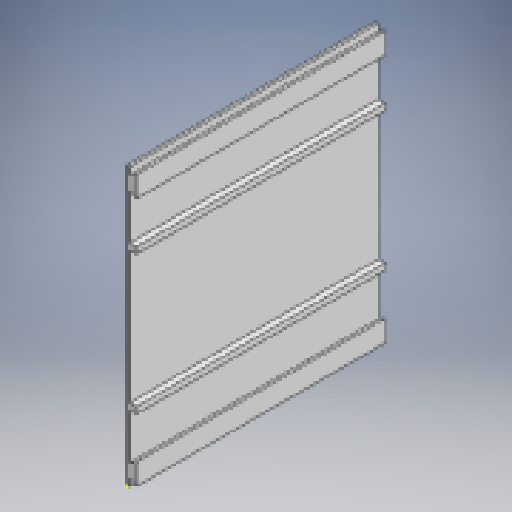
# Autodesk Inventor part: side
Saved by Autodesk Inventor 2025.2 (Build 292293000, 293)
## iProperties
Created: 2025-02-22
Part Number: side
Material: Generic
Document SubType Name: Modeling
Designer: email
Density: 1 g/cm^3
Appearance: Default
Author: email
Autodesk Inventor part; units mm, degrees
ref_plane "YZ Plane" through (0, 0, 0) normal (1, 0, 0) x (0, 1, 0)
ref_plane "XZ Plane" through (0, 0, 0) normal (0, 1, 0) x (-1, 0, 0)
ref_plane "XY Plane" through (0, 0, 0) normal (0, 0, 1) x (1, 0, 0)
sketch "Sketch1" plane through (0, 0, 0) normal (0, 0, 1) x (1, 0, 0)
  line L0 (0, 0) -> (0, 100)
  line L1 (0, 100) -> (1, 100)
  line L2 (1, 100) -> (1, 97.5)
  line L3 (1, 97.5) -> (3.5, 99)
  line L4 (3.5, 99) -> (3.5, 91)
  line L5 (3.5, 91) -> (1, 92.5)
  line L6 (1, 92.5) -> (1, 7.5)
  line L7 (1, 7.5) -> (3.5, 9)
  line L8 (3.5, 9) -> (3.5, 1)
  line L9 (3.5, 1) -> (1, 2.5)
  line L10 (1, 2.5) -> (1, 0)
  line L11 (1, 0) -> (0, 0)
  line L12 (1, 76.25) -> (3.5, 76.25)
  line L13 (3.5, 76.25) -> (3.5, 73.75)
  line L14 (3.5, 73.75) -> (1, 73.75)
  line L15 (1, 73.75) -> (1, 76.25)
  line L16 (1, 23.75) -> (3.5, 23.75)
  line L17 (3.5, 23.75) -> (3.5, 26.25)
  line L18 (3.5, 26.25) -> (1, 26.25)
  line L19 (1, 26.25) -> (1, 23.75)
  line L20 (3.4, 98.8234) -> (0.9, 97.3234)
  line L21 (0.9, 97.3234) -> (0.9, 99.9)
  line L22 (0.9, 99.9) -> (0.1, 99.9)
  line L23 (0.1, 99.9) -> (0.1, 0.1)
  line L24 (0.1, 0.1) -> (0.9, 0.1)
  line L25 (0.9, 0.1) -> (0.9, 2.6766)
  line L26 (0.9, 2.6766) -> (3.4, 1.1766)
  line L27 (3.4, 1.1766) -> (3.4, 8.8234)
  line L28 (3.4, 8.8234) -> (0.9, 7.3234)
  line L29 (0.9, 7.3234) -> (0.9, 92.6766)
  line L30 (0.9, 92.6766) -> (3.4, 91.1766)
  line L31 (3.4, 91.1766) -> (3.4, 98.8234)
  line L32 (1, 92.5) -> (1, 97.5)
  line L33 (1, 2.5) -> (1, 7.5)
  point P0 (1, 98.75)
  point P1 (0.5, 0)
  point P2 (3.5, 75)
  point P3 (3.5, 25)
  point P4 (1, 97.3834)
  point P5 (1, 92.6166)
  point P6 (1, 7.3834)
  point P7 (1, 2.6166)
  dimension "d0" = 8
  dimension "d1" = 8
  dimension "d2" = 2.5
  dimension "d3" = 2.5
  dimension "d4" = 1
  dimension "d5" = 1
  dimension "d6" = 100
  dimension "d7" = 5
  dimension "d8" = 5
  dimension "d10" = 2.5
  dimension "d11" = 7.5
  dimension "d12" = 2.5
  dimension "d13" = 1
  dimension "d16" = 2.5
  dimension "d17" = 2.5
  dimension "d18" = 2.5
  dimension "d19" = 2.5
  dimension "d20" = 25
  dimension "d21" = 25
  dimension "d24" = 0.1
  constraints: 68 end point, 13 parallel, 5 point on line, 4 midpoint, 4 perpendicular, 4 vertical, 2 collinear, 2 horizontal, 11 other
  measures "d0" distance of L3.end L4.end
  measures "d1" distance of L7.end L8.end
  measures "d2" distance between parallel lines of L6 L8
  measures "d3" distance from line of point (1, 98.75) L4
  measures "d4" distance from line of L1 L3.end
  measures "d5" vertical distance of point (0.5, 0) L8.end
  measures "d6" distance of L0.start L0.end
  measures "d7" distance of L5.end L2.end
  measures "d8" distance of L6.end L9.end
  measures "d10" distance of L1.end L2.end
  measures "d11" distance of L1.end L5.end
  measures "d12" distance of L10.end L9.end
  measures "d13" distance between parallel lines of L0 L6
  measures "d16" distance between parallel lines of L6 L13
  measures "d17" distance between parallel lines of L19 L17
  measures "d18" distance between parallel lines of L16 L18
  measures "d19" distance between parallel lines of L14 L12
  measures "d20" distance from line of L1 point (3.5, 75)
  measures "d21" distance from line of L11 point (3.5, 25)
  measures "d24" distance between parallel lines of L3 L20
extrude "Extrusion1" add sketch "Sketch1" along normal blind 90 contours L0 L1 L2 L32 L20 L21 L22 L23 L24 L25 L26 L33 L10 L11 | L33 L26 L27 L28 L7 L8 L9 | L3 L4 L5 L32 L30 L31 L20 | L33 L28 L27 L26 | L26 L25 L24 L23 L22 L21 L20 L32 L30 L29 L28 L33 | L20 L31 L30 L32 | L28 L29 L30 L32 L6 L33
extrude "Extrusion2" add sketch "Sketch1" along normal blind 90 contours L6 L18 L17 L16 | L12 L13 L14 L6
ref_plane "Work Plane1" through (0, 0, 90) normal (0, 0, -1) x (0, 1, 0)
extrude "Extrusion3" cut sketch "Sketch1" along normal up to surface (90 mm away) contours L33 L26 L27 L28 L7 L8 L9 | L3 L4 L5 L32 L30 L31 L20
sketch "Sketch2" plane through (0, 0, 90) normal (0, 0, 1) x (1, 0, 0)
  point P0 (0, 0)
sketch "Sketch3" plane through (0, 0, 90) normal (0, 0, 1) x (1, 0, 0)
  line L0 (1, 97.3834) -> (1, 100) projected
  line L1 (1, 100) -> (0, 100) projected
  line L2 (0, 100) -> (0, 0) projected
  line L3 (0, 0) -> (1, 0) projected
  line L4 (1, 0) -> (1, 2.6166) projected
  line L5 (1, 2.6166) -> (3.4, 1.1766) projected
  line L6 (3.4, 1.1766) -> (3.4, 8.8234) projected
  line L7 (3.4, 8.8234) -> (1, 7.3834) projected
  line L8 (1, 7.3834) -> (1, 23.75) projected
  line L9 (1, 23.75) -> (3.5, 23.75) projected
  line L10 (3.5, 23.75) -> (3.5, 26.25) projected
  line L11 (3.5, 26.25) -> (1, 26.25) projected
  line L12 (1, 26.25) -> (1, 73.75) projected
  line L13 (1, 73.75) -> (3.5, 73.75) projected
  line L14 (3.5, 73.75) -> (3.5, 76.25) projected
  line L15 (3.5, 76.25) -> (1, 76.25) projected
  line L16 (1, 76.25) -> (1, 92.6166) projected
  line L17 (1, 92.6166) -> (3.4, 91.1766) projected
  line L18 (3.4, 91.1766) -> (3.4, 98.8234) projected
  line L19 (3.4, 98.8234) -> (1, 97.3834) projected
extrude "Extrusion4" cut sketch "Sketch3" against normal blind 0.1
sketch "Sketch4" plane through (0, 0, 0) normal (0, 0, -1) x (-1, 0, 0)
  line L0 (-3.5, 76.25) -> (-1, 76.25) projected
  line L1 (-3.5, 73.75) -> (-3.5, 76.25) projected
  line L2 (-1, 73.75) -> (-3.5, 73.75) projected
  line L3 (-3.5, 26.25) -> (-1, 26.25) projected
  line L4 (-3.5, 23.75) -> (-3.5, 26.25) projected
  line L5 (-1, 23.75) -> (-3.5, 23.75) projected
  line L6 (-1, 76.15) -> (-3.4, 76.15)
  line L7 (-3.4, 76.15) -> (-3.4, 73.85)
  line L8 (-3.4, 73.85) -> (-1, 73.85)
  line L9 (-1, 26.15) -> (-3.4, 26.15)
  line L10 (-3.4, 26.15) -> (-3.4, 23.85)
  line L11 (-3.4, 23.85) -> (-1, 23.85)
  line L12 (-1, 76.25) -> (-1, 73.75)
  line L13 (-1, 26.25) -> (-1, 23.75)
  point P0 (0, 0)
  dimension "d29" = 0.1
  dimension "tol" = 0.1
  constraints: 16 end point, 1 collinear, 1 vertical, 4 other
  measures "d29" distance between parallel lines of L0 L6
  measures "tol" distance between parallel lines of L3 L9
extrude "Extrusion5" cut sketch "Sketch4" against normal through all contours L0 L12 L6 L7 L8 L2 L1 | L3 L13 L9 L10 L11 L5 L4
equation "\"d27\" = tol"
equation "\"d29\" = tol"
body "Solid1"
